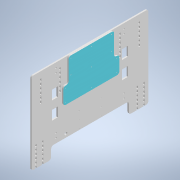
# Autodesk Inventor part: Platforma_kolesa
Saved by Autodesk Inventor 2021.1 (Build 251245010, 245A)
## iProperties
Created: 2023-02-16
Part Number: Platforma_kolesa
Material: Типовые
Document SubType Name: Modeling
Designer: User
Density: 1 g/cm^3
Appearance: По умолчанию
Author: User
Autodesk Inventor part; units mm, degrees
ref_plane "YZ Plane" through (0, 0, 0) normal (1, 0, 0) x (0, 1, 0)
ref_plane "XZ Plane" through (0, 0, 0) normal (0, 1, 0) x (-1, 0, 0)
ref_plane "РабПлоскость1" through (-17.9787, -14.0323, 120.6673) normal (-1, 0, 0) x (0, -1, 0)
sketch "Эскиз1" plane through (-17.9787, -14.0323, 120.6673) normal (-1, 0, 0) x (0, -1, 0)
  line L0 (229.7011, 135.6275) -> (-110.2989, 135.6275)
  line L1 (-110.2989, 135.6275) -> (-110.2989, -364.3725)
  line L2 (-110.2989, -364.3725) -> (229.7011, -364.3725)
  arc A0 (-82.855, -357.465) -> (-82.855, -332.065) centre (-51.0789, -344.765) ccw construction
  line L3 (-57, -322.88) -> (-67, -322.88) projected
  line L4 (-67, -322.88) -> (-67, -328.88) projected
  line L5 (-57, -328.88) -> (-67, -328.88) projected
  line L6 (-57, -322.88) -> (-57, -328.88) projected
  line L7 (-73, -322.88) -> (-83, -322.88) projected
  line L8 (-83, -322.88) -> (-83, -328.88) projected
  line L9 (-73, -328.88) -> (-83, -328.88) projected
  line L10 (-73, -322.88) -> (-73, -328.88) projected
  line L11 (-40, -322.88) -> (-50, -322.88) projected
  line L12 (-50, -322.88) -> (-50, -328.88) projected
  line L13 (-40, -328.88) -> (-50, -328.88) projected
  line L14 (-40, -322.88) -> (-40, -328.88) projected
  line L15 (-23, -322.88) -> (-33, -322.88) projected
  line L16 (-33, -322.88) -> (-33, -328.88) projected
  line L17 (-23, -328.88) -> (-33, -328.88) projected
  line L18 (-23, -322.88) -> (-23, -328.88) projected
  line L19 (-6, -322.88) -> (-16, -322.88) projected
  line L20 (-16, -322.88) -> (-16, -328.88) projected
  line L21 (-6, -328.88) -> (-16, -328.88) projected
  line L22 (-6, -322.88) -> (-6, -328.88) projected
  line L23 (10, -322.88) -> (0, -322.88) projected
  line L24 (0, -322.88) -> (0, -328.88) projected
  line L25 (10, -328.88) -> (0, -328.88) projected
  line L26 (10, -322.88) -> (10, -328.88) projected
  line L27 (10, -245.88) -> (0, -245.88) projected
  line L28 (10, -245.88) -> (10, -239.88) projected
  line L29 (10, -239.88) -> (0, -239.88) projected
  line L30 (0, -245.88) -> (0, -239.88) projected
  line L31 (-6, -245.88) -> (-16, -245.88) projected
  line L32 (-6, -245.88) -> (-6, -239.88) projected
  line L33 (-6, -239.88) -> (-16, -239.88) projected
  line L34 (-16, -245.88) -> (-16, -239.88) projected
  line L35 (-23, -245.88) -> (-33, -245.88) projected
  line L36 (-23, -245.88) -> (-23, -239.88) projected
  line L37 (-23, -239.88) -> (-33, -239.88) projected
  line L38 (-33, -245.88) -> (-33, -239.88) projected
  line L39 (-40, -245.88) -> (-50, -245.88) projected
  line L40 (-40, -245.88) -> (-40, -239.88) projected
  line L41 (-40, -239.88) -> (-50, -239.88) projected
  line L42 (-50, -245.88) -> (-50, -239.88) projected
  line L43 (-57, -245.88) -> (-67, -245.88) projected
  line L44 (-57, -245.88) -> (-57, -239.88) projected
  line L45 (-57, -239.88) -> (-67, -239.88) projected
  line L46 (-67, -245.88) -> (-67, -239.88) projected
  line L47 (-73, -245.88) -> (-83, -245.88) projected
  line L48 (-73, -245.88) -> (-73, -239.88) projected
  line L49 (-73, -239.88) -> (-83, -239.88) projected
  line L50 (-83, -245.88) -> (-83, -239.88) projected
  line L51 (64.7011, -114.3725) -> (-110.2989, -114.3725) construction
  line L52 (-57, 94.1349) -> (-67, 94.1349)
  line L53 (-67, 94.1349) -> (-67, 100.1349)
  line L54 (-57, 100.1349) -> (-67, 100.1349)
  line L55 (-57, 94.1349) -> (-57, 100.1349)
  line L56 (-73, 94.1349) -> (-83, 94.1349)
  line L57 (-83, 94.1349) -> (-83, 100.1349)
  line L58 (-73, 100.1349) -> (-83, 100.1349)
  line L59 (-73, 94.1349) -> (-73, 100.1349)
  line L60 (-40, 94.1349) -> (-50, 94.1349)
  line L61 (-50, 94.1349) -> (-50, 100.1349)
  line L62 (-40, 100.1349) -> (-50, 100.1349)
  line L63 (-40, 94.1349) -> (-40, 100.1349)
  line L64 (-23, 94.1349) -> (-33, 94.1349)
  line L65 (-33, 94.1349) -> (-33, 100.1349)
  line L66 (-23, 100.1349) -> (-33, 100.1349)
  line L67 (-23, 94.1349) -> (-23, 100.1349)
  line L68 (-6, 94.1349) -> (-16, 94.1349)
  line L69 (-16, 94.1349) -> (-16, 100.1349)
  line L70 (-6, 100.1349) -> (-16, 100.1349)
  line L71 (-6, 94.1349) -> (-6, 100.1349)
  line L72 (10, 94.1349) -> (0, 94.1349)
  line L73 (0, 94.1349) -> (0, 100.1349)
  line L74 (10, 100.1349) -> (0, 100.1349)
  line L75 (10, 94.1349) -> (10, 100.1349)
  line L76 (10, 17.1349) -> (0, 17.1349)
  line L77 (10, 17.1349) -> (10, 11.1349)
  line L78 (10, 11.1349) -> (0, 11.1349)
  line L79 (0, 17.1349) -> (0, 11.1349)
  line L80 (-6, 17.1349) -> (-16, 17.1349)
  line L81 (-6, 17.1349) -> (-6, 11.1349)
  line L82 (-6, 11.1349) -> (-16, 11.1349)
  line L83 (-16, 17.1349) -> (-16, 11.1349)
  line L84 (-23, 17.1349) -> (-33, 17.1349)
  line L85 (-23, 17.1349) -> (-23, 11.1349)
  line L86 (-23, 11.1349) -> (-33, 11.1349)
  line L87 (-33, 17.1349) -> (-33, 11.1349)
  line L88 (-40, 17.1349) -> (-50, 17.1349)
  line L89 (-40, 17.1349) -> (-40, 11.1349)
  line L90 (-40, 11.1349) -> (-50, 11.1349)
  line L91 (-50, 17.1349) -> (-50, 11.1349)
  line L92 (-57, 17.1349) -> (-67, 17.1349)
  line L93 (-57, 17.1349) -> (-57, 11.1349)
  line L94 (-57, 11.1349) -> (-67, 11.1349)
  line L95 (-67, 17.1349) -> (-67, 11.1349)
  line L96 (-73, 17.1349) -> (-83, 17.1349)
  line L97 (-73, 17.1349) -> (-73, 11.1349)
  line L98 (-73, 11.1349) -> (-83, 11.1349)
  line L99 (-83, 17.1349) -> (-83, 11.1349)
  arc A1 (-100.2989, 135.6275) -> (-110.2989, 125.6275) centre (-100.2989, 125.6275) ccw
  arc A2 (189.7011, 125.6275) -> (179.7011, 135.6275) centre (179.7011, 125.6275) ccw
  line L100 (0, -328.88) -> (-6, -328.88) construction
  circle A3 centre (-3, -325.88) radius 1.5
  line L101 (0, -245.88) -> (-6, -245.88) construction
  line L102 (0, -245.88) -> (0, -239.88)
  line L103 (0, -242.88) -> (-6, -242.88) construction
  line L104 (-16, -328.88) -> (-23, -328.88) construction
  line L105 (-19.5, -328.88) -> (-19.5, -322.88) construction
  line L106 (-3, -328.88) -> (-3, -322.88) construction
  circle A4 centre (-3, -242.88) radius 1.5
  circle A5 centre (-19.5, -242.88) radius 1.5
  circle A6 centre (-19.5, -325.88) radius 1.5
  line L107 (-50, -328.88) -> (-57, -328.88) construction
  line L108 (-67, -328.88) -> (-73, -328.88) construction
  line L109 (-50, -245.88) -> (-57, -245.88) construction
  line L110 (-73, -245.88) -> (-67, -245.88) construction
  circle A7 centre (-53.5, -242.88) radius 1.5
  circle A8 centre (-70, -242.88) radius 1.5
  circle A9 centre (-53.5, -325.88) radius 1.5
  circle A10 centre (-70, -325.88) radius 1.5
  arc A11 (-110.2989, -354.3725) -> (-100.2989, -364.3725) centre (-100.2989, -354.3725) ccw
  circle A12 centre (-3, 97.1349) radius 1.5
  circle A13 centre (-3, 14.1349) radius 1.5
  circle A14 centre (-19.5, 14.1349) radius 1.5
  circle A15 centre (-19.5, 97.1349) radius 1.5
  circle A16 centre (-53.5, 97.1349) radius 1.5
  circle A17 centre (-53.5, 14.1349) radius 1.5
  circle A18 centre (-70, 97.1349) radius 1.5
  circle A19 centre (-70, 14.1349) radius 1.5
  line L111 (189.7011, 42.0519) -> (189.7011, -270.797)
  line L112 (239.7011, 68.4849) -> (239.7011, 52.0519)
  line L113 (239.7011, 52.0519) -> (199.7011, 52.0519)
  arc A20 (239.7011, 125.6275) -> (229.7011, 135.6275) centre (229.7011, 125.6275) ccw
  arc A21 (229.7011, 52.0519) -> (239.7011, 62.0519) centre (229.7011, 62.0519) ccw
  line L114 (239.7011, -280.797) -> (199.7011, -280.797)
  arc A22 (239.7011, -290.797) -> (229.7011, -280.797) centre (229.7011, -290.797) ccw
  arc A23 (229.7011, -364.3725) -> (239.7011, -354.3725) centre (229.7011, -354.3725) ccw
  arc A24 (199.7011, 52.0519) -> (189.7011, 42.0519) centre (199.7011, 42.0519) ccw
  arc A25 (189.7011, -270.797) -> (199.7011, -280.797) centre (199.7011, -270.797) ccw
  arc A26 (189.7011, 125.6275) -> (179.7011, 135.6275) centre (179.7011, 125.6275) ccw
  line L115 (239.7011, -354.3725) -> (239.7011, -290.797)
  line L116 (239.7011, 125.6275) -> (239.7011, 68.4849)
  line L117 (230.9213, -341.94) -> (240.9213, -341.94) projected
  line L118 (230.9213, -341.94) -> (230.9213, -347.94) projected
  line L119 (230.9213, -347.94) -> (240.9213, -347.94) projected
  line L120 (240.9213, -341.94) -> (240.9213, -347.94) projected
  line L121 (230.9213, -347.94) -> (240.9213, -347.94)
  line L122 (240.9213, -347.94) -> (240.9213, -341.94)
  line L123 (240.9213, -341.94) -> (230.9213, -341.94)
  line L124 (230.9213, -341.94) -> (230.9213, -347.94)
  line L125 (150.9213, -319.94) -> (160.9213, -319.94) projected
  line L126 (160.9213, -319.94) -> (160.9213, -313.94) projected
  line L127 (150.9213, -313.94) -> (160.9213, -313.94) projected
  line L128 (150.9213, -319.94) -> (150.9213, -313.94) projected
  line L129 (214.9213, -341.94) -> (214.9213, -347.94)
  line L130 (214.9213, -347.94) -> (224.9213, -347.94)
  line L131 (224.9213, -347.94) -> (224.9213, -341.94)
  line L132 (224.9213, -341.94) -> (214.9213, -341.94)
  line L133 (198.9213, -341.94) -> (198.9213, -347.94)
  line L134 (198.9213, -347.94) -> (208.9213, -347.94)
  line L135 (208.9213, -347.94) -> (208.9213, -341.94)
  line L136 (208.9213, -341.94) -> (198.9213, -341.94)
  line L137 (182.9213, -341.94) -> (182.9213, -347.94)
  line L138 (182.9213, -347.94) -> (192.9213, -347.94)
  line L139 (192.9213, -347.94) -> (192.9213, -341.94)
  line L140 (192.9213, -341.94) -> (182.9213, -341.94)
  line L141 (166.9213, -341.94) -> (166.9213, -347.94)
  line L142 (166.9213, -347.94) -> (176.9213, -347.94)
  line L143 (176.9213, -347.94) -> (176.9213, -341.94)
  line L144 (176.9213, -341.94) -> (166.9213, -341.94)
  line L145 (150.9213, -341.94) -> (150.9213, -347.94)
  line L146 (150.9213, -347.94) -> (160.9213, -347.94)
  line L147 (160.9213, -347.94) -> (160.9213, -341.94)
  line L148 (160.9213, -341.94) -> (150.9213, -341.94)
  line L149 (230.9213, -313.94) -> (230.9213, -319.94)
  line L150 (230.9213, -319.94) -> (240.9213, -319.94)
  line L151 (240.9213, -319.94) -> (240.9213, -313.94)
  line L152 (240.9213, -313.94) -> (230.9213, -313.94)
  line L153 (214.9213, -313.94) -> (214.9213, -319.94)
  line L154 (214.9213, -319.94) -> (224.9213, -319.94)
  line L155 (224.9213, -319.94) -> (224.9213, -313.94)
  line L156 (224.9213, -313.94) -> (214.9213, -313.94)
  line L157 (198.9213, -313.94) -> (198.9213, -319.94)
  line L158 (198.9213, -319.94) -> (208.9213, -319.94)
  line L159 (208.9213, -319.94) -> (208.9213, -313.94)
  line L160 (208.9213, -313.94) -> (198.9213, -313.94)
  line L161 (182.9213, -313.94) -> (182.9213, -319.94)
  line L162 (182.9213, -319.94) -> (192.9213, -319.94)
  line L163 (192.9213, -319.94) -> (192.9213, -313.94)
  line L164 (192.9213, -313.94) -> (182.9213, -313.94)
  line L165 (166.9213, -313.94) -> (166.9213, -319.94)
  line L166 (166.9213, -319.94) -> (176.9213, -319.94)
  line L167 (176.9213, -319.94) -> (176.9213, -313.94)
  line L168 (176.9213, -313.94) -> (166.9213, -313.94)
  line L169 (150.9213, -313.94) -> (150.9213, -319.94)
  line L170 (150.9213, -319.94) -> (160.9213, -319.94)
  line L171 (160.9213, -319.94) -> (160.9213, -313.94)
  line L172 (160.9213, -313.94) -> (150.9213, -313.94)
  circle A27 centre (227.9213, -344.94) radius 1.5
  circle A28 centre (211.9213, -344.94) radius 1.5
  circle A29 centre (195.9213, -344.94) radius 1.5
  circle A30 centre (179.9213, -344.94) radius 1.5
  circle A31 centre (163.9213, -344.94) radius 1.5
  circle A32 centre (227.9213, -316.94) radius 1.5
  circle A33 centre (211.9213, -316.94) radius 1.5
  circle A34 centre (195.9213, -316.94) radius 1.5
  circle A35 centre (179.9213, -316.94) radius 1.5
  circle A36 centre (163.9213, -316.94) radius 1.5
  line L173 (230.9213, 113.1949) -> (240.9213, 113.1949)
  line L174 (230.9213, 113.1949) -> (230.9213, 119.1949)
  line L175 (230.9213, 119.1949) -> (240.9213, 119.1949)
  line L176 (240.9213, 113.1949) -> (240.9213, 119.1949)
  line L177 (230.9213, 119.1949) -> (240.9213, 119.1949)
  line L178 (240.9213, 119.1949) -> (240.9213, 113.1949)
  line L179 (240.9213, 113.1949) -> (230.9213, 113.1949)
  line L180 (230.9213, 113.1949) -> (230.9213, 119.1949)
  line L181 (150.9213, 91.1949) -> (160.9213, 91.1949)
  line L182 (160.9213, 91.1949) -> (160.9213, 85.1949)
  line L183 (150.9213, 85.1949) -> (160.9213, 85.1949)
  line L184 (150.9213, 91.1949) -> (150.9213, 85.1949)
  line L185 (214.9213, 113.1949) -> (214.9213, 119.1949)
  line L186 (214.9213, 119.1949) -> (224.9213, 119.1949)
  line L187 (224.9213, 119.1949) -> (224.9213, 113.1949)
  line L188 (224.9213, 113.1949) -> (214.9213, 113.1949)
  line L189 (198.9213, 113.1949) -> (198.9213, 119.1949)
  line L190 (198.9213, 119.1949) -> (208.9213, 119.1949)
  line L191 (208.9213, 119.1949) -> (208.9213, 113.1949)
  line L192 (208.9213, 113.1949) -> (198.9213, 113.1949)
  line L193 (182.9213, 113.1949) -> (182.9213, 119.1949)
  line L194 (182.9213, 119.1949) -> (192.9213, 119.1949)
  line L195 (192.9213, 119.1949) -> (192.9213, 113.1949)
  line L196 (192.9213, 113.1949) -> (182.9213, 113.1949)
  line L197 (166.9213, 113.1949) -> (166.9213, 119.1949)
  line L198 (166.9213, 119.1949) -> (176.9213, 119.1949)
  line L199 (176.9213, 119.1949) -> (176.9213, 113.1949)
  line L200 (176.9213, 113.1949) -> (166.9213, 113.1949)
  line L201 (150.9213, 113.1949) -> (150.9213, 119.1949)
  line L202 (150.9213, 119.1949) -> (160.9213, 119.1949)
  line L203 (160.9213, 119.1949) -> (160.9213, 113.1949)
  line L204 (160.9213, 113.1949) -> (150.9213, 113.1949)
  line L205 (230.9213, 85.1949) -> (230.9213, 91.1949)
  line L206 (230.9213, 91.1949) -> (240.9213, 91.1949)
  line L207 (240.9213, 91.1949) -> (240.9213, 85.1949)
  line L208 (240.9213, 85.1949) -> (230.9213, 85.1949)
  line L209 (214.9213, 85.1949) -> (214.9213, 91.1949)
  line L210 (214.9213, 91.1949) -> (224.9213, 91.1949)
  line L211 (224.9213, 91.1949) -> (224.9213, 85.1949)
  line L212 (224.9213, 85.1949) -> (214.9213, 85.1949)
  line L213 (198.9213, 85.1949) -> (198.9213, 91.1949)
  line L214 (198.9213, 91.1949) -> (208.9213, 91.1949)
  line L215 (208.9213, 91.1949) -> (208.9213, 85.1949)
  line L216 (208.9213, 85.1949) -> (198.9213, 85.1949)
  line L217 (182.9213, 85.1949) -> (182.9213, 91.1949)
  line L218 (182.9213, 91.1949) -> (192.9213, 91.1949)
  line L219 (192.9213, 91.1949) -> (192.9213, 85.1949)
  line L220 (192.9213, 85.1949) -> (182.9213, 85.1949)
  line L221 (166.9213, 85.1949) -> (166.9213, 91.1949)
  line L222 (166.9213, 91.1949) -> (176.9213, 91.1949)
  line L223 (176.9213, 91.1949) -> (176.9213, 85.1949)
  line L224 (176.9213, 85.1949) -> (166.9213, 85.1949)
  line L225 (150.9213, 85.1949) -> (150.9213, 91.1949)
  line L226 (150.9213, 91.1949) -> (160.9213, 91.1949)
  line L227 (160.9213, 91.1949) -> (160.9213, 85.1949)
  line L228 (160.9213, 85.1949) -> (150.9213, 85.1949)
  circle A37 centre (227.9213, 116.1949) radius 1.5
  circle A38 centre (211.9213, 116.1949) radius 1.5
  circle A39 centre (195.9213, 116.1949) radius 1.5
  circle A40 centre (179.9213, 116.1949) radius 1.5
  circle A41 centre (163.9213, 116.1949) radius 1.5
  circle A42 centre (227.9213, 88.1949) radius 1.5
  circle A43 centre (211.9213, 88.1949) radius 1.5
  circle A44 centre (195.9213, 88.1949) radius 1.5
  circle A45 centre (179.9213, 88.1949) radius 1.5
  circle A46 centre (163.9213, 88.1949) radius 1.5
  point P0 (-14.0323, -120.6673)
  point P1 (239.7011, -364.3725)
  point P2 (-82.855, 103.3199)
  point P3 (239.7011, -114.3725)
  point P4 (239.7011, -1.355)
  point P5 (239.7011, -244.525)
  point P6 (189.7011, 52.0519)
  point P7 (189.7011, -280.797)
  point P8 (229.7011, 125.6275)
  point P9 (150.9213, -316.94)
  point P10 (155.9213, -313.94)
  point P11 (150.9213, 88.1949)
  point P12 (155.9213, 85.1949)
  point P13 (239.7011, 85.1949)
  point P14 (239.7011, 91.1949)
  point P15 (239.7011, 113.1949)
  point P16 (239.7011, 119.1949)
  point P17 (239.7011, -347.94)
  point P18 (239.7011, -341.94)
  point P19 (239.7011, -319.94)
  point P20 (239.7011, -313.94)
  dimension "d0" = 350
  dimension "d1" = 500
  dimension "d2" = 59.22
  dimension "d4" = 10
  dimension "d7" = 10
  dimension "d21" = 3
  dimension "d30" = 3
  dimension "d31" = 3
  dimension "d32" = 3
  dimension "d33" = 3
  dimension "d34" = 3
  dimension "d35" = 3
  dimension "d36" = 3
  dimension "d37" = 10
  dimension "d47" = 3
  dimension "d48" = 3
  dimension "d49" = 3
  dimension "d50" = 3
  dimension "d51" = 3
  dimension "d52" = 3
  dimension "d53" = 3
  dimension "d54" = 3
  dimension "d76" = 10
  dimension "d77" = 10
  dimension "d78" = 10
  dimension "d118" = 16
  dimension "d121" = 28
  dimension "d124" = 3
  dimension "d127" = 16
  dimension "d130" = 28
  constraints: 346 end point, 121 symmetric about line, 47 centre point, 23 point on circle, 13 midpoint, 13 point on line, 12 tangent, 6 horizontal, 6 vertical, 5 collinear, 4 parallel, 4 perpendicular, 1 coincident, 1 equal radius, 122 other
  measures "d0" distance of point (239.701, -364.373) L1.end
  measures "d1" distance of L1.end L0.end
  measures "d2" distance from line of L1 A0.centre
  measures "d4" radius of A1
  measures "d7" radius of A2
  measures "d21" diameter of A3
  measures "d30" diameter of A4
  measures "d31" diameter of A5
  measures "d32" diameter of A6
  measures "d33" diameter of A7
  measures "d34" diameter of A8
  measures "d35" diameter of A9
  measures "d36" diameter of A10
  measures "d37" radius of A11
  measures "d47" diameter of A12
  measures "d48" diameter of A13
  measures "d49" diameter of A14
  measures "d50" diameter of A15
  measures "d51" diameter of A16
  measures "d52" diameter of A17
  measures "d53" diameter of A18
  measures "d54" diameter of A19
  measures "d76" radius of A20
  measures "d77" radius of A21
  measures "d78" radius of A23
  measures "d118" distance of L123.end L129.start
  measures "d121" distance of L123.end L149.start
  measures "d124" diameter of A27
  measures "d127" distance of A27.centre A28.centre
  measures "d130" distance of A27.centre A32.centre
ref_plane "РабПлоскость2" through (-11.9787, 52.9677, 197.6673) normal (-1, 0, 0) x (0, 0, 1)
extrude "Выдавливание1" add sketch "Эскиз1" against normal up to surface (6 mm away) contours A20 L116 L175 L174 L173 L206 L205 L208 L112 A21 L113 A24 L111 A25 L114 A22 L115 L152 L149 L150 L117 L118 L119 A23 L2 A11 L1 A1 L0
sketch "Эскиз2" plane through (-17.9787, -14.0323, 120.6673) normal (-1, 0, 0) x (0, 0, 1)
  line L0 (48.1275, -57.2011) -> (48.1275, -97.2011) projected
  line L1 (-1.8725, -57.2011) -> (-1.8725, -97.2011) projected
  line L2 (23.1275, -57.2011) -> (48.1275, -57.2011)
  line L3 (48.1275, -97.2011) -> (23.1275, -97.2011) projected
  line L4 (-251.8725, -22.2011) -> (-276.8725, -22.2011) projected
  line L5 (23.1275, -57.2011) -> (48.1275, -57.2011)
  line L6 (48.1275, -22.2011) -> (23.1275, -22.2011) projected
  line L7 (-251.8725, -57.2011) -> (-251.8725, -97.2011) projected
  line L8 (-251.8725, -97.2011) -> (-276.8725, -97.2011) projected
  line L9 (-276.8725, -97.2011) -> (-276.8725, -57.2011) projected
  line L10 (-276.8725, -57.2011) -> (-251.8725, -57.2011) projected
  line L11 (-251.8725, 17.7989) -> (-251.8725, -22.2011) projected
  line L12 (-276.8725, -22.2011) -> (-276.8725, 17.7989) projected
  line L13 (-276.8725, 17.7989) -> (-251.8725, 17.7989) projected
  line L14 (48.1275, -57.2011) -> (48.1275, -97.2011) projected
  line L15 (23.1275, -22.2011) -> (23.1275, 17.7989) projected
  line L16 (23.1275, 17.7989) -> (48.1275, 17.7989) projected
  line L17 (48.1275, 17.7989) -> (48.1275, -22.2011) projected
  line L18 (-354.3725, -189.7011) -> (125.6275, -189.7011) projected
  arc A0 (125.6275, -189.7011) -> (135.6275, -179.7011) centre (125.6275, -179.7011) ccw projected
  line L19 (135.6275, -179.7011) -> (135.6275, 100.2989) projected
  arc A1 (135.6275, 100.2989) -> (125.6275, 110.2989) centre (125.6275, 100.2989) ccw projected
  line L20 (125.6275, 110.2989) -> (-354.3725, 110.2989) projected
  arc A2 (-354.3725, 110.2989) -> (-364.3725, 100.2989) centre (-354.3725, 100.2989) ccw projected
  line L21 (-364.3725, 100.2989) -> (-364.3725, -179.7011) projected
  arc A3 (-364.3725, -179.7011) -> (-354.3725, -189.7011) centre (-354.3725, -179.7011) ccw projected
  circle A4 centre (10.6275, -4.7011) radius 2.5 projected
  circle A5 centre (-94.3725, -179.7011) radius 2.5 projected
  circle A6 centre (-94.3725, -153.9868) radius 2.5 projected
  circle A7 centre (-94.3725, -128.2725) radius 2.5 projected
  circle A8 centre (-94.3725, -102.5582) radius 2.5 projected
  circle A9 centre (-134.3725, -89.7011) radius 2.5 projected
  circle A10 centre (-134.3725, -115.4154) radius 2.5 projected
  circle A11 centre (-134.3725, -141.1296) radius 2.5 projected
  circle A12 centre (-134.3725, -166.8439) radius 2.5 projected
  circle A13 centre (-134.3725, -179.7011) radius 2.5 projected
  circle A14 centre (-301.8725, -39.7011) radius 2 projected
  circle A15 centre (-176.8725, -39.7011) radius 2 projected
  circle A16 centre (-51.8725, -39.7011) radius 2 projected
  circle A17 centre (73.1275, -39.7011) radius 2 projected
  circle A18 centre (-114.3725, -114.7011) radius 2 projected
  circle A19 centre (-114.3725, 35.2989) radius 2 projected
  circle A20 centre (-134.3725, -153.9868) radius 2.5 projected
  circle A21 centre (-134.3725, -128.2725) radius 2.5 projected
  circle A22 centre (-134.3725, -102.5582) radius 2.5 projected
  circle A23 centre (-94.3725, -89.7011) radius 2.5 projected
  circle A24 centre (-94.3725, -115.4154) radius 2.5 projected
  circle A25 centre (-94.3725, -141.1296) radius 2.5 projected
  circle A26 centre (-94.3725, -166.8439) radius 2.5 projected
  circle A27 centre (-239.3725, -4.7011) radius 2.5 projected
  line L22 (-117.3725, 87.7989) -> (-111.3725, 87.7989) projected
  line L23 (-111.3725, 87.7989) -> (-111.3725, 57.7989) projected
  line L24 (-111.3725, 57.7989) -> (-117.3725, 57.7989) projected
  line L25 (-117.3725, 57.7989) -> (-117.3725, 87.7989) projected
  line L26 (-117.3725, 12.7989) -> (-111.3725, 12.7989) projected
  line L27 (-111.3725, 12.7989) -> (-111.3725, -17.2011) projected
  line L28 (-111.3725, -17.2011) -> (-117.3725, -17.2011) projected
  line L29 (-117.3725, -17.2011) -> (-117.3725, 12.7989) projected
  line L30 (-117.3725, -62.2011) -> (-111.3725, -62.2011) projected
  line L31 (-111.3725, -62.2011) -> (-111.3725, -92.2011) projected
  line L32 (-111.3725, -92.2011) -> (-117.3725, -92.2011) projected
  line L33 (-117.3725, -92.2011) -> (-117.3725, -62.2011) projected
  line L34 (-117.3725, -137.2011) -> (-111.3725, -137.2011) projected
  line L35 (-111.3725, -137.2011) -> (-111.3725, -167.2011) projected
  line L36 (-111.3725, -167.2011) -> (-117.3725, -167.2011) projected
  line L37 (-117.3725, -167.2011) -> (-117.3725, -137.2011) projected
  line L38 (119.3775, -42.7011) -> (89.3775, -42.7011) projected
  line L39 (89.3775, -42.7011) -> (89.3775, -36.7011) projected
  line L40 (89.3775, -36.7011) -> (119.3775, -36.7011) projected
  line L41 (119.3775, -36.7011) -> (119.3775, -42.7011) projected
  line L42 (56.8775, -42.7011) -> (26.8775, -42.7011) projected
  line L43 (26.8775, -42.7011) -> (26.8775, -36.7011) projected
  line L44 (26.8775, -36.7011) -> (56.8775, -36.7011) projected
  line L45 (56.8775, -36.7011) -> (56.8775, -42.7011) projected
  line L46 (-5.6225, -42.7011) -> (-35.6225, -42.7011) projected
  line L47 (-35.6225, -42.7011) -> (-35.6225, -36.7011) projected
  line L48 (-35.6225, -36.7011) -> (-5.6225, -36.7011) projected
  line L49 (-5.6225, -36.7011) -> (-5.6225, -42.7011) projected
  line L50 (-68.1225, -42.7011) -> (-98.1225, -42.7011) projected
  line L51 (-98.1225, -42.7011) -> (-98.1225, -36.7011) projected
  line L52 (-98.1225, -36.7011) -> (-68.1225, -36.7011) projected
  line L53 (-68.1225, -36.7011) -> (-68.1225, -42.7011) projected
  line L54 (-130.6225, -42.7011) -> (-160.6225, -42.7011) projected
  line L55 (-160.6225, -42.7011) -> (-160.6225, -36.7011) projected
  line L56 (-160.6225, -36.7011) -> (-130.6225, -36.7011) projected
  line L57 (-130.6225, -36.7011) -> (-130.6225, -42.7011) projected
  line L58 (-193.1225, -42.7011) -> (-223.1225, -42.7011) projected
  line L59 (-223.1225, -42.7011) -> (-223.1225, -36.7011) projected
  line L60 (-223.1225, -36.7011) -> (-193.1225, -36.7011) projected
  line L61 (-193.1225, -36.7011) -> (-193.1225, -42.7011) projected
  line L62 (-255.6225, -42.7011) -> (-285.6225, -42.7011) projected
  line L63 (-285.6225, -42.7011) -> (-285.6225, -36.7011) projected
  line L64 (-285.6225, -36.7011) -> (-255.6225, -36.7011) projected
  line L65 (-255.6225, -36.7011) -> (-255.6225, -42.7011) projected
  line L66 (-348.1225, -36.7011) -> (-318.1225, -36.7011) projected
  line L67 (-318.1225, -36.7011) -> (-318.1225, -42.7011) projected
  line L68 (-318.1225, -42.7011) -> (-348.1225, -42.7011) projected
  line L69 (-348.1225, -42.7011) -> (-348.1225, -36.7011) projected
  line L70 (23.1275, -97.2011) -> (23.1275, -57.2011)
  circle A28 centre (31.4028, 89.4418) radius 3 projected
  circle A29 centre (31.4028, 70.7916) radius 3 projected
  circle A30 centre (31.4028, -150.1937) radius 3 projected
  circle A31 centre (31.4028, -168.8439) radius 3 projected
  circle A32 centre (-260.1478, -168.8439) radius 3 projected
  circle A33 centre (-260.1478, -150.1937) radius 3 projected
  circle A34 centre (-260.1478, 70.7916) radius 3 projected
  circle A35 centre (-260.1478, 89.4418) radius 3 projected
  point P0 (-120.6673, 14.0323)
  constraints: 6 end point, 1 vertical
extrude "Выдавливание2" cut sketch "Эскиз2" against normal blind 6 contours L0 L3 L70 L2 | L4 L12 L13 L11 | L6 L15 L16 L17 | L7 L8 L9 L10 | A28 | A29 | A30 | A31 | A32 | A33 | A34 | A35
sketch "Эскиз3" plane through (-11.9787, -243.7333, -243.7053) normal (1, 0, 0) x (0, 0, -1)
  circle A0 centre (-353, 55) radius 5.75
  circle A1 centre (-297.5, 111.5) radius 1.6 projected
  circle A2 centre (-297.5, 79) radius 1.6 projected
  circle A3 centre (-297.5, 46) radius 1.6 projected
  circle A4 centre (-202.5, 46) radius 1.6 projected
  circle A5 centre (-202.5, 79) radius 1.6 projected
  circle A6 centre (-202.5, 111.5) radius 1.6 projected
  line L0 (-303, 40) -> (-303, 138.5) projected
  line L1 (-10, 40) -> (-490, 40) projected
  point P0 (-243.7053, 243.7333)
  dimension "d98" = 11.5
  dimension "d171" = 50
  dimension "d172" = 15
  constraints: 1 centre point
  measures "d98" diameter of A0
  measures "d171" distance from line of L0 A0.centre
  measures "d172" distance from line of L1 A0.centre
extrude "Выдавливание3" cut sketch "Эскиз3" against normal blind 6
sketch "Эскиз5" plane through (-11.9787, -243.7333, -243.7053) normal (1, 0, 0) x (0, 0, -1)
  line L0 (-93.5755, 40) -> (-406.4245, 40)
  line L1 (-406.4245, 40) -> (-93.5755, 40)
  line L2 (-140.4925, 239.8781) -> (-142.8435, 239.8781)
  line L3 (-152.8435, 249.8781) -> (-152.8435, 330)
  line L4 (-490, 340) -> (-10, 340)
  line L5 (-359.5075, 239.8781) -> (-357.1565, 239.8781)
  line L6 (-347.1565, 249.8781) -> (-347.1565, 330)
  circle A0 centre (-162.8435, 330) radius 1.5
  circle A1 centre (-162.8435, 268) radius 1.5
  circle A2 centre (-140.4925, 178) radius 1.5
  line L7 (-369.5075, 229.8781) -> (-369.5075, 178)
  line L8 (-359.5075, 168) -> (-303.4899, 168)
  line L9 (-130.4925, 229.8781) -> (-130.4925, 178)
  circle A3 centre (-140.4925, 229.8781) radius 1.5
  arc A4 (-140.4925, 168) -> (-130.4925, 178) centre (-140.4925, 178) ccw
  arc A5 (-130.4925, 229.8781) -> (-140.4925, 239.8781) centre (-140.4925, 229.8781) ccw
  arc A6 (-152.8435, 249.8781) -> (-142.8435, 239.8781) centre (-142.8435, 249.8781) ccw
  line L10 (-162.8435, 340) -> (-337.1565, 340)
  arc A7 (-337.1565, 340) -> (-347.1565, 330) centre (-337.1565, 330) ccw
  arc A8 (-152.8435, 330) -> (-162.8435, 340) centre (-162.8435, 330) ccw
  arc A9 (-357.1565, 239.8781) -> (-347.1565, 249.8781) centre (-357.1565, 249.8781) ccw
  arc A10 (-359.5075, 239.8781) -> (-369.5075, 229.8781) centre (-359.5075, 229.8781) ccw
  arc A11 (-369.5075, 178) -> (-359.5075, 168) centre (-359.5075, 178) ccw
  line L11 (-162.8435, 330) -> (-162.8435, 340)
  line L12 (-142.8435, 252.7822) -> (-142.8435, 276.1742)
  line L13 (-124.4925, 223.7011) -> (-124.4925, 219.7011)
  line L14 (-357.1565, 279.547) -> (-357.1565, 256.1549)
  line L15 (-375.5075, 223.6281) -> (-375.5075, 231.8608)
  line L16 (-259.79, 162) -> (-208, 162)
  line L17 (-118.4925, 245.9511) -> (-124.4925, 245.9511)
  line L18 (-381.5075, 245.8781) -> (-375.5075, 245.8781)
  line L19 (-140.4925, 168) -> (-359.5075, 168)
  line L20 (-250, 168) -> (-250, 340) construction
  circle A12 centre (-337.1565, 330) radius 1.5
  circle A13 centre (-337.1565, 268) radius 1.5
  circle A14 centre (-359.5075, 178) radius 1.5
  circle A15 centre (-359.5075, 229.8781) radius 1.5
  line L21 (-337.1565, 330) -> (-337.1565, 340)
  circle A16 centre (-250, 178) radius 1.5
  circle A17 centre (-250, 254) radius 1.5
  circle A18 centre (-250, 330) radius 1.5
  point P0 (-130.4925, 239.8781)
  point P1 (-152.8435, 239.8781)
  point P2 (-152.8435, 340)
  point P3 (-368.0534, 40)
  point P4 (-369.5075, 239.8781)
  point P5 (-347.1565, 239.8781)
  point P6 (-347.1565, 340)
  point P7 (-369.5075, 168)
  point P8 (-130.4925, 168)
  point P9 (-337.1565, 340)
extrude "Выдавливание4" add sketch "Эскиз5" along normal blind 6 separate body
sketch "Эскиз6" plane through (-11.9787, -243.7333, -243.7053) normal (1, 0, 0) x (0, 0, -1)
  arc A0 (-337.1565, 340) -> (-347.1565, 330) centre (-337.1565, 330) ccw projected
  line L0 (-347.1565, 330) -> (-347.1565, 249.8781) projected
  arc A1 (-357.1565, 239.8781) -> (-347.1565, 249.8781) centre (-357.1565, 249.8781) ccw projected
  line L1 (-357.1565, 239.8781) -> (-359.5075, 239.8781) projected
  arc A2 (-359.5075, 239.8781) -> (-369.5075, 229.8781) centre (-359.5075, 229.8781) ccw projected
  line L2 (-369.5075, 229.8781) -> (-369.5075, 178) projected
  arc A3 (-369.5075, 178) -> (-359.5075, 168) centre (-359.5075, 178) ccw projected
  arc A4 (-140.4925, 168) -> (-130.4925, 178) centre (-140.4925, 178) ccw projected
  line L3 (-130.4925, 178) -> (-130.4925, 229.8781) projected
  arc A5 (-130.4925, 229.8781) -> (-140.4925, 239.8781) centre (-140.4925, 229.8781) ccw projected
  line L4 (-140.4925, 239.8781) -> (-142.8435, 239.8781) projected
  arc A6 (-152.8435, 249.8781) -> (-142.8435, 239.8781) centre (-142.8435, 249.8781) ccw projected
  line L5 (-152.8435, 249.8781) -> (-152.8435, 330) projected
  arc A7 (-152.8435, 330) -> (-162.8435, 340) centre (-162.8435, 330) ccw projected
  circle A8 centre (-162.8435, 330) radius 1.5 projected
  circle A9 centre (-140.4925, 229.8781) radius 1.5 projected
  circle A10 centre (-162.8435, 268) radius 1.5 projected
  circle A11 centre (-140.4925, 178) radius 1.5 projected
  line L6 (-359.5075, 168) -> (-140.4925, 168) projected
  line L7 (-162.8435, 340) -> (-337.1565, 340) projected
  point P0 (-243.7053, 243.7333)
extrude "Выдавливание5" cut sketch "Эскиз6" against normal blind 6 contours A8 | A9 | A10 | A11 bodies 1
